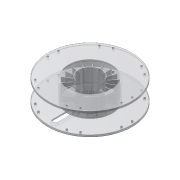
# Autodesk Inventor part: filament spool
Saved by Autodesk Inventor 2015 (Build 190159000, 159)
## iProperties
Created: 2018-06-07
Part Number: filament spool
Material: Generic
Document SubType Name: Modeling
Designer: Ghassan Yusuf
Density: 1 g/cm^3
Appearance: Clear(1)
Author: Ghassan Yusuf
Autodesk Inventor part; units mm, degrees
ref_plane "YZ Plane" through (0, 0, 0) normal (1, 0, 0) x (0, 1, 0)
ref_plane "XZ Plane" through (0, 0, 0) normal (0, 1, 0) x (-1, 0, 0)
ref_plane "XY Plane" through (0, 0, 0) normal (0, 0, 1) x (1, 0, 0)
sketch "filament spool drawing" plane through (0, 0, 0) normal (0, 0, 1) x (1, 0, 0)
  circle A0 centre (0, 0) radius 100
  circle A1 centre (0, 0) radius 26
  circle A2 centre (0, 0) radius 28.75
  circle A3 centre (0, 0) radius 50.5
  circle A4 centre (0, 0) radius 53.25
  dimension "d0" = 200
  dimension "d1" = 52
  dimension "d2" = 2.75
  dimension "d3" = 101
  dimension "d4" = 2.75
  measures "d0" diameter of A0
  measures "d1" diameter of A1
  measures "d2" radial gap between concentric circles of A1 A2
  measures "d3" diameter of A3
  measures "d4" radial gap between concentric circles of A3 A4
sketch "Sketch1" plane through (0, 0, 0) normal (0, 0, 1) x (1, 0, 0)
  circle A0 centre (0, 0) radius 100
  circle A1 centre (0, 0) radius 26
  circle A2 centre (0, 0) radius 28.75
  circle A3 centre (0, 0) radius 50.5
  circle A4 centre (0, 0) radius 53.25
  constraints: 1 other
extrude "Extrusion1" add sketch "Sketch1" along normal mid plane 54 contours A0 | A2 | A3 | A4
sketch "Sketch2" plane through (0, 0, 0) normal (0, 0, 1) x (1, 0, 0)
  circle A0 centre (0, 0) radius 100
  circle A1 centre (0, 0) radius 26
  circle A2 centre (0, 0) radius 28.75
  circle A3 centre (0, 0) radius 50.5
  circle A4 centre (0, 0) radius 53.25
  constraints: 1 other
extrude "Extrusion2" cut sketch "Sketch2" along normal mid plane 44 contours A0
sketch "Sketch3" plane through (0, 0, 27) normal (0, 0, 1) x (1, 0, 0)
  circle A0 centre (0, 0) radius 100
  circle A1 centre (0, 0) radius 26
  circle A2 centre (0, 0) radius 28.75
  circle A3 centre (0, 0) radius 50.5
  circle A4 centre (0, 0) radius 53.25
  constraints: 1 other
extrude "Extrusion3" cut sketch "Sketch3" against normal blind 8.7 contours A3
extrude "Extrusion4" add sketch "Sketch3" along normal blind 2 contours A2
sketch "Sketch4" plane through (0, 0, -27) normal (0, 0, -1) x (-1, 0, 0)
  circle A0 centre (0, 0) radius 100
  circle A1 centre (0, 0) radius 26
  circle A2 centre (0, 0) radius 28.75
  circle A3 centre (0, 0) radius 50.5
  circle A4 centre (0, 0) radius 53.25
  constraints: 1 other
extrude "Extrusion5" add sketch "Sketch4" along normal blind 2.6 contours A2
sketch "Sketch5" plane through (0, 0, -27) normal (0, 0, -1) x (-1, 0, 0)
  line L0 (6, -89) -> (-6, -89)
  line L1 (-6, -89) -> (-6, -37)
  line L2 (-6, -37) -> (6, -37)
  line L3 (6, -37) -> (6, -89)
  arc A0 (6, -43) -> (-6, -43) centre (0, -43) ccw
  arc A1 (-6, -83) -> (6, -83) centre (0, -83) ccw
  point P0 (0, 0)
  point P1 (0, -37)
  dimension "d15" = 12
  dimension "d16" = 52
  dimension "d17" = 37
  constraints: 8 end point, 4 point on circle, 4 point on line, 4 tangent, 2 centre point, 2 parallel, 1 horizontal, 1 midpoint, 1 perpendicular, 1 vertical alignment
  measures "d15" distance of L1.end L2.end
  measures "d16" distance of L0.end L1.end
  measures "d17" distance from line of point (0, 0) L2
extrude "Extrusion6" cut sketch "Sketch5" against normal blind 5 contours A1 L1 A0 L3
sketch "Sketch6" plane through (0, 0, -27) normal (0, 0, -1) x (-1, 0, 0)
  circle A0 centre (-31.654, -86.9686) radius 2.15
  circle A1 centre (0, 0) radius 100
  circle A2 centre (0, 0) radius 92.55
  circle A3 centre (-53.1998, -75.7317) radius 2.15
  line L0 (0, 0) -> (-31.654, -86.9686)
  line L1 (0, 0) -> (110, 0) construction
  circle A4 centre (59.49, -70.8974) radius 2.15
  circle A5 centre (38.9857, -83.9382) radius 2.15
  circle A6 centre (91.144, 16.0711) radius 2.15
  circle A7 centre (92.1854, -8.2065) radius 2.15
  circle A8 centre (31.654, 86.9686) radius 2.15
  circle A9 centre (53.1998, 75.7317) radius 2.15
  circle A10 centre (-59.49, 70.8974) radius 2.15
  circle A11 centre (-38.9857, 83.9382) radius 2.15
  circle A12 centre (-91.144, -16.0711) radius 2.15
  circle A13 centre (-92.1854, 8.2065) radius 2.15
  dimension "d20" = 4.3
  dimension "d21" = 7.45
  dimension "d22" = 24.3
  dimension "d24" = 110
  dimension "d27" = 360
  constraints: 14 centre point, 4 end point, 2 point on circle, 1 coincident, 1 equal radius, 1 horizontal, 25 other
  measures "d20" diameter of A0
  measures "d21" radial gap between concentric circles of A1 A2
  measures "d22" distance of L0.end A3.centre
  measures "d24" angle of L0 L1
extrude "Extrusion7" cut sketch "Sketch6" against normal blind 74.5 contours A0 A2 L0 | L0 A2 A0 | A0 A2 | A5 A2 | A2 A5 | A3 A2 | A2 A3 | A4 A2 | A2 A4 | A12 A2 | A2 A12 | A7 A2 | A2 A7 | A13 A2 | A2 A13 | A10 A2 | A2 A10 | A6 A2 | A2 A6 | A11 A2 | A2 A11 | A9 A2 | A2 A9 | A8 A2 | A2 A8
fillet "Fillet1" radius 0.6 7 edges at (-100, 0, 27) (-100, 0, 22) (-100, 0, -22) (-100, 0, -27) (-50.5, 0, 27) (-28.75, 0, 29) (-26, 0, 29)
sketch "Sketch7" plane through (0, 0, 18.3) normal (0, 0, 1) x (1, 0, 0)
  circle A0 centre (0, 0) radius 51.1 projected
  circle A1 centre (0, 0) radius 28.15 projected
  arc A2 (0.75, 28.7402) -> (-0.75, 28.7402) centre (0, 0) ccw
  arc A3 (0.75, 50.4944) -> (-0.75, 50.4944) centre (0, 0) ccw
  line L0 (-0.75, 51.1) -> (-0.75, 51.0945)
  line L1 (-0.75, 50.4944) -> (-0.75, 28.7402)
  line L2 (0.75, 28.7402) -> (0.75, 50.4944)
  line L3 (0.75, 51.0945) -> (0.75, 51.1)
  circle A4 centre (0, 0) radius 50.5 projected
  circle A5 centre (0, 0) radius 28.75 projected
  arc A6 (-9.125, 27.2635) -> (-10.5345, 26.7505) centre (0, 0) ccw
  arc A7 (-16.5653, 47.7058) -> (-17.9749, 47.1927) centre (0, 0) ccw
  line L4 (-18.182, 47.7618) -> (-18.1801, 47.7566)
  line L5 (-17.9749, 47.1927) -> (-10.5345, 26.7505)
  line L6 (-9.125, 27.2635) -> (-16.5653, 47.7058)
  line L7 (-16.7706, 48.2696) -> (-16.7725, 48.2748)
  arc A8 (-17.8993, 22.4984) -> (-19.0484, 21.5342) centre (0, 0) ccw
  arc A9 (-31.8827, 39.1631) -> (-33.0317, 38.1989) centre (0, 0) ccw
  line L8 (-33.421, 38.6628) -> (-33.4174, 38.6586)
  line L9 (-33.0317, 38.1989) -> (-19.0484, 21.5342)
  line L10 (-17.8993, 22.4984) -> (-31.8827, 39.1631)
  line L11 (-32.2684, 39.6227) -> (-32.2719, 39.627)
  arc A10 (-24.5148, 15.0196) -> (-25.2648, 13.7206) centre (0, 0) ccw
  arc A11 (-43.3545, 25.8967) -> (-44.1045, 24.5977) centre (0, 0) ccw
  line L12 (-44.6289, 24.9005) -> (-44.6241, 24.8977)
  line L13 (-44.1045, 24.5977) -> (-25.2648, 13.7206)
  line L14 (-24.5148, 15.0196) -> (-43.3545, 25.8967)
  line L15 (-43.8741, 26.1968) -> (-43.8789, 26.1995)
  arc A12 (-28.1734, 5.7293) -> (-28.4338, 4.2521) centre (0, 0) ccw
  arc A13 (-49.5971, 9.5069) -> (-49.8575, 8.0297) centre (0, 0) ccw
  line L16 (-50.4539, 8.1348) -> (-50.4485, 8.1339)
  line L17 (-49.8575, 8.0297) -> (-28.4338, 4.2521)
  line L18 (-28.1734, 5.7293) -> (-49.5971, 9.5069)
  line L19 (-50.188, 9.6111) -> (-50.1934, 9.612)
  arc A14 (-28.4338, -4.2521) -> (-28.1734, -5.7293) centre (0, 0) ccw
  arc A15 (-49.8575, -8.0297) -> (-49.5971, -9.5069) centre (0, 0) ccw
  line L20 (-50.1934, -9.612) -> (-50.188, -9.6111)
  line L21 (-49.5971, -9.5069) -> (-28.1734, -5.7293)
  line L22 (-28.4338, -4.2521) -> (-49.8575, -8.0297)
  line L23 (-50.4485, -8.1339) -> (-50.4539, -8.1348)
  arc A16 (-25.2648, -13.7206) -> (-24.5148, -15.0196) centre (0, 0) ccw
  arc A17 (-44.1045, -24.5977) -> (-43.3545, -25.8967) centre (0, 0) ccw
  line L24 (-43.8789, -26.1995) -> (-43.8741, -26.1968)
  line L25 (-43.3545, -25.8967) -> (-24.5148, -15.0196)
  line L26 (-25.2648, -13.7206) -> (-44.1045, -24.5977)
  line L27 (-44.6241, -24.8977) -> (-44.6289, -24.9005)
  arc A18 (-19.0484, -21.5342) -> (-17.8993, -22.4984) centre (0, 0) ccw
  arc A19 (-33.0317, -38.1989) -> (-31.8827, -39.1631) centre (0, 0) ccw
  line L28 (-32.2719, -39.627) -> (-32.2684, -39.6227)
  line L29 (-31.8827, -39.1631) -> (-17.8993, -22.4984)
  line L30 (-19.0484, -21.5342) -> (-33.0317, -38.1989)
  line L31 (-33.4174, -38.6586) -> (-33.421, -38.6628)
  arc A20 (-10.5345, -26.7505) -> (-9.125, -27.2635) centre (0, 0) ccw
  arc A21 (-17.9749, -47.1927) -> (-16.5653, -47.7058) centre (0, 0) ccw
  line L32 (-16.7725, -48.2748) -> (-16.7706, -48.2696)
  line L33 (-16.5653, -47.7058) -> (-9.125, -27.2635)
  line L34 (-10.5345, -26.7505) -> (-17.9749, -47.1927)
  line L35 (-18.1801, -47.7566) -> (-18.182, -47.7618)
  arc A22 (-0.75, -28.7402) -> (0.75, -28.7402) centre (0, 0) ccw
  arc A23 (-0.75, -50.4944) -> (0.75, -50.4944) centre (0, 0) ccw
  line L36 (0.75, -51.1) -> (0.75, -51.0945)
  line L37 (0.75, -50.4944) -> (0.75, -28.7402)
  line L38 (-0.75, -28.7402) -> (-0.75, -50.4944)
  line L39 (-0.75, -51.0945) -> (-0.75, -51.1)
  arc A24 (9.125, -27.2635) -> (10.5345, -26.7505) centre (0, 0) ccw
  arc A25 (16.5653, -47.7058) -> (17.9749, -47.1927) centre (0, 0) ccw
  line L40 (18.182, -47.7618) -> (18.1801, -47.7566)
  line L41 (17.9749, -47.1927) -> (10.5345, -26.7505)
  line L42 (9.125, -27.2635) -> (16.5653, -47.7058)
  line L43 (16.7706, -48.2696) -> (16.7725, -48.2748)
  arc A26 (17.8993, -22.4984) -> (19.0484, -21.5342) centre (0, 0) ccw
  arc A27 (31.8827, -39.1631) -> (33.0317, -38.1989) centre (0, 0) ccw
  line L44 (33.421, -38.6628) -> (33.4174, -38.6586)
  line L45 (33.0317, -38.1989) -> (19.0484, -21.5342)
  line L46 (17.8993, -22.4984) -> (31.8827, -39.1631)
  line L47 (32.2684, -39.6227) -> (32.2719, -39.627)
  arc A28 (24.5148, -15.0196) -> (25.2648, -13.7206) centre (0, 0) ccw
  arc A29 (43.3545, -25.8967) -> (44.1045, -24.5977) centre (0, 0) ccw
  line L48 (44.6289, -24.9005) -> (44.6241, -24.8977)
  line L49 (44.1045, -24.5977) -> (25.2648, -13.7206)
  line L50 (24.5148, -15.0196) -> (43.3545, -25.8967)
  line L51 (43.8741, -26.1968) -> (43.8789, -26.1995)
  arc A30 (28.1734, -5.7293) -> (28.4338, -4.2521) centre (0, 0) ccw
  arc A31 (49.5971, -9.5069) -> (49.8575, -8.0297) centre (0, 0) ccw
  line L52 (50.4539, -8.1348) -> (50.4485, -8.1339)
  line L53 (49.8575, -8.0297) -> (28.4338, -4.2521)
  line L54 (28.1734, -5.7293) -> (49.5971, -9.5069)
  line L55 (50.188, -9.6111) -> (50.1934, -9.612)
  arc A32 (28.4338, 4.2521) -> (28.1734, 5.7293) centre (0, 0) ccw
  arc A33 (49.8575, 8.0297) -> (49.5971, 9.5069) centre (0, 0) ccw
  line L56 (50.1934, 9.612) -> (50.188, 9.6111)
  line L57 (49.5971, 9.5069) -> (28.1734, 5.7293)
  line L58 (28.4338, 4.2521) -> (49.8575, 8.0297)
  line L59 (50.4485, 8.1339) -> (50.4539, 8.1348)
  arc A34 (25.2648, 13.7206) -> (24.5148, 15.0196) centre (0, 0) ccw
  arc A35 (44.1045, 24.5977) -> (43.3545, 25.8967) centre (0, 0) ccw
  line L60 (43.8789, 26.1995) -> (43.8741, 26.1968)
  line L61 (43.3545, 25.8967) -> (24.5148, 15.0196)
  line L62 (25.2648, 13.7206) -> (44.1045, 24.5977)
  line L63 (44.6241, 24.8977) -> (44.6289, 24.9005)
  arc A36 (19.0484, 21.5342) -> (17.8993, 22.4984) centre (0, 0) ccw
  arc A37 (33.0317, 38.1989) -> (31.8827, 39.1631) centre (0, 0) ccw
  line L64 (32.2719, 39.627) -> (32.2684, 39.6227)
  line L65 (31.8827, 39.1631) -> (17.8993, 22.4984)
  line L66 (19.0484, 21.5342) -> (33.0317, 38.1989)
  line L67 (33.4174, 38.6586) -> (33.421, 38.6628)
  arc A38 (10.5345, 26.7505) -> (9.125, 27.2635) centre (0, 0) ccw
  arc A39 (17.9749, 47.1927) -> (16.5653, 47.7058) centre (0, 0) ccw
  line L68 (16.7725, 48.2748) -> (16.7706, 48.2696)
  line L69 (16.5653, 47.7058) -> (9.125, 27.2635)
  line L70 (10.5345, 26.7505) -> (17.9749, 47.1927)
  line L71 (18.1801, 47.7566) -> (18.182, 47.7618)
  dimension "d33" = 1.5
  dimension "d36" = 360
  constraints: 144 end point, 74 point on circle, 36 centre point, 19 coincident, 4 parallel, 2 concentric, 289 other
  measures "d33" distance between parallel lines of L2 L1
extrude "Extrusion8" cut sketch "Sketch7" against normal blind 40.3 contours L2 A4 L69 A5 | A5 L6 A4 L1 | L70 A4 L65 A5 | A5 L10 A4 L5 | L66 A4 L61 A5 | A5 L14 A4 L9 | L62 A4 L57 A5 | A5 L18 A4 L13 | L58 A4 L53 A5 | A5 L22 A4 L17 | A5 L26 A4 L21 | L54 A4 L49 A5 | A5 L30 A4 L25 | L50 A4 L45 A5 | A5 L34 A4 L29 | L46 A4 L41 A5 | A5 L38 A4 L33 | L42 A4 L37 A5
sketch "Sketch8" plane through (0, 0, -27) normal (0, 0, -1) x (-1, 0, 0)
  arc A0 (6, -43) -> (-6, -43) centre (0, -43) ccw
  arc A1 (-6, -50.1423) -> (6, -50.1423) centre (0, 0) ccw
  line L0 (-6, -43) -> (-6, -50.1423)
  arc A2 (-0.75, -37.0471) -> (-6, -43) centre (0, -43) ccw projected
  line L1 (-6, -50.1423) -> (-6, -43) projected
  line L2 (6, -43) -> (6, -50.1423)
  line L3 (6, -43) -> (6, -50.1423) projected
  point P0 (0, 0)
  point P1 (0.75, -37.0471)
  constraints: 5 point on circle, 4 end point, 2 centre point, 2 collinear, 1 tangent
extrude "Extrusion9" cut sketch "Sketch8" against normal blind 83.05
sketch "Sketch9" plane through (0, 0, -22) normal (0, 0, 1) x (1, 0, 0)
  arc A0 (6, -43) -> (-6, -43) centre (0, -43) ccw
  arc A1 (-6, -50.1423) -> (6, -50.1423) centre (0, 0) ccw
  line L0 (-6, -43) -> (-6, -50.1423)
  arc A2 (-0.75, -37.0471) -> (-6, -43) centre (0, -43) ccw projected
  line L1 (-6, -43) -> (-6, -83) projected
  line L2 (6, -43) -> (6, -50.1423)
  line L3 (6, -50.1423) -> (6, -43) projected
  arc A3 (7.5, -43) -> (-7.5, -43) centre (0, -43) ccw
  line L4 (7.5, -43) -> (7.5, -51.4563)
  arc A4 (-7.5, -51.4563) -> (7.5, -51.4563) centre (0, 0) ccw
  line L5 (-7.5, -51.4563) -> (-7.5, -43)
  point P0 (0, 0)
  dimension "d42" = 1.5
  constraints: 9 point on circle, 8 end point, 4 centre point, 2 collinear, 1 tangent, 3 other
  measures "d42" radial gap between concentric circles of A0 A3
extrude "Extrusion10" add sketch "Sketch9" along normal blind 40.3
chamfer "Chamfer1" distance 2 angle 45 6 edges at (6, -46.5711, -27) (6, -66.5711, -27) (0, -37, -27) (-6, -46.5711, -27) (-6, -66.5711, -27) (0, -89, -27)
body "Solid1"
